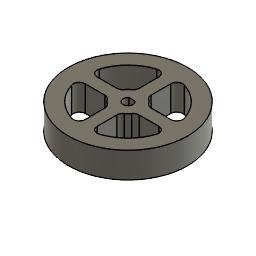
GIC wheels (Autodesk Fusion 360 design; units mm, degrees)
Autodesk Fusion 360 part; units mm, degrees
sketch "Sketch1" plane through (0, 0, 0) normal (0, 1, 0) x (1, 0, 0)
  circle A0 centre (0, 0) radius 2.5
  spline S0 degree 5 poles (-1.8, 2) (-1.648, 2) (-1.344, 2) (-0.888, 2) (-0.28, 2) (0.48, 2) (1.088, 2) (1.544, 2) (1.848, 2) (2, 2) knots 0 0 0 0 0 0 0.2 0.4 0.6 0.8 1 1 1 1 1 1
  circle A1 centre (0, 0) radius 4
  dimension "d1" = 5
  dimension "d2" = 8
  constraint coincident A0.centre A1.centre
  measures "d1" diameter of A0
  measures "d2" diameter of A1
extrude "Extrude1" add sketch "Sketch1" along normal blind 25 contours A0 S0 | A1 picked at (0.3999, 2.0645)
sketch "Sketch2" plane through (0, 25, 0) normal (0, 1, 0) x (-1, 0, 0)
  arc A0 (1.5, -2) -> (-1.5, -2) centre (0, 0) ccw
  line L0 (1.5, -2) -> (-1.5, -2)
  circle A1 centre (0, 0) radius 4
  circle A2 centre (0, 0) radius 30
  dimension "d5" = 60
  constraint coincident A0.centre A1.centre
  measures "d5" diameter of A2
extrude "Extrude2" add sketch "Sketch2" against normal blind 15 contours A2
sketch "Sketch3" plane through (0, 25, 0) normal (0, 1, 0) x (-1, 0, 0)
  circle A0 centre (0, 0) radius 30
  arc A1 (1.5, -2) -> (-1.5, -2) centre (0, 0) ccw
  line L0 (1.5, -2) -> (-1.5, -2)
  line L1 (3, -25) -> (-3, -25)
  line L2 (-3, -25) -> (-3, 23)
  line L3 (-3, 23) -> (3, 23)
  line L4 (3, 23) -> (3, -25)
  line L5 (26, -3) -> (-27, -3)
  line L6 (-27, -3) -> (-27, 3)
  line L7 (-27, 3) -> (26, 3)
  line L8 (26, 3) -> (26, -3)
  circle A2 centre (0, 0) radius 7.5
  circle A3 centre (0, 0) radius 22.5
  dimension "d8" = 15
  dimension "d9" = 45
  constraint horizontal L1
  constraint vertical L2
  constraint horizontal L3
  constraint vertical L4
  constraint horizontal L5
  constraint vertical L6
  constraint horizontal L7
  constraint vertical L8
  constraint coincident A0.centre A1.centre
  measures "d8" diameter of A2
  measures "d9" diameter of A3
extrude "Extrude3" cut sketch "Sketch3" against normal blind 27 contours L4 L5 A2 A3 | L2 L5 A2 A3 | L2 L7 A2 A3 | L4 L7 A2 A3
fillet "Fillet1" radius 3 16 edges at (22.2991, 17.5, -3) (3, 17.5, -22.2991) (-3, 17.5, -22.2991) (-22.2991, 17.5, -3) (-22.2991, 17.5, 3) (-3, 17.5, 22.2991) (3, 17.5, 22.2991) (22.2991, 17.5, 3) (3, 17.5, 6.8739) (6.8739, 17.5, 3) (-6.8739, 17.5, 3) (-3, 17.5, 6.8739) (-6.8739, 17.5, -3) (-3, 17.5, -6.8739) (3, 17.5, -6.8739) (6.8739, 17.5, -3)
extrude "Extrude4" cut 1 faces at (0.0996, 0, -2.6629) along direction (0, 1, 0) blind 2
extrude "Extrude5" cut 1 faces at (-0.7473, 10, 23.8692) along direction (0, 1, 0) blind 2
fillet "Fillet2" radius 2 1 edges at (-3.7293, 12, -1.4465)
